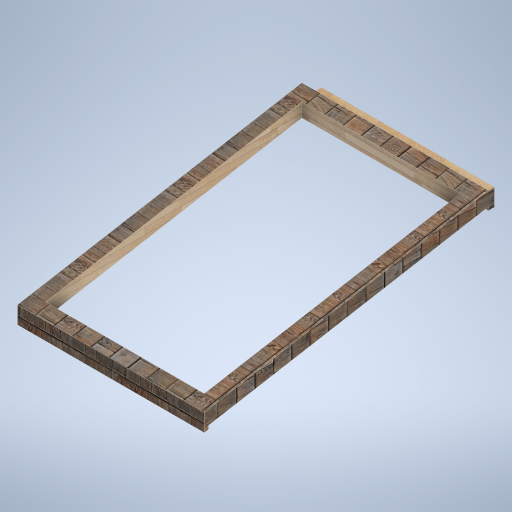
# Autodesk Inventor part: eave_frame_01
Saved by Autodesk Inventor 2024.3 (Build 283343000, 343)
## iProperties
Created: 2024-05-23
Part Number: eave_frame_01
Material: Wood (Maple)
Document SubType Name: Modeling
Designer: Huang
Density: 0.67 g/cm^3
Appearance: Natural Maple - Glossy Dark Tint
Author: Huang
Autodesk Inventor part; units mm, degrees
ref_plane "YZ Plane" through (0, 0, 0) normal (1, 0, 0) x (0, 1, 0)
ref_plane "XZ Plane" through (0, 0, 0) normal (0, 1, 0) x (-1, 0, 0)
sketch "Sketch19" plane through (0, 0, 0) normal (0, 0, 1) x (1, 0, 0)
  line L0 (1200.9555, -1496.1779) -> (1200.9555, 1503.8221)
  line L1 (-4726.1559, 1503.8221) -> (4728.0669, 1503.8221)
  line L2 (4418.0669, -1496.1779) -> (4418.0669, 1503.8221)
  line L3 (1200.9555, 1503.8221) -> (4418.0669, 1503.8221)
  line L4 (1200.9555, 1503.8221) -> (1000.9555, 1503.8221)
  line L5 (1000.9555, 1503.8221) -> (1000.9555, -1496.1779)
  line L6 (2809.5112, 1503.8221) -> (2609.5112, 1503.8221)
  line L7 (2609.5112, 1503.8221) -> (2609.5112, -1496.1779)
  line L8 (2609.5112, -1496.1779) -> (2509.5112, -1496.1779)
  line L9 (2509.5112, -1496.1779) -> (2509.5112, 1503.8221)
  line L10 (1200.9555, -1496.1779) -> (1000.9555, -1496.1779)
  line L11 (1000.9555, 1503.8221) -> (1000.9555, 1353.8221)
  line L12 (1000.9555, 1353.8221) -> (2609.5112, 1353.8221)
  point P0 (0, 0)
  dimension "d29" = 200
  dimension "d30" = 200
  dimension "d31" = 100
  dimension "d32" = 150
  constraints: 26 end point, 6 perpendicular, 5 point on line, 2 coincident, 1 collinear, 1 midpoint
  measures "d29" distance of L3.start L4.end
  measures "d30" distance of L6.start L6.end
  measures "d31" distance of L7.end L8.end
  measures "d32" distance of L4.end L11.end
ref_plane "Work Plane17" through (0, 0, 2500) normal (0, 0, 1) x (1, 0, 0)
sketch "Sketch20" plane through (0, 0, 2500) normal (0, 0, 1) x (1, 0, 0)
  line L0 (-4726.1559, 1503.8221) -> (4728.0669, 1503.8221) projected
  line L1 (1200.9555, -1496.1779) -> (1200.9555, 1503.8221) projected
  line L2 (1000.9555, 1503.8221) -> (1000.9555, -1496.1779) projected
  line L3 (2509.5112, -1496.1779) -> (2509.5112, 1503.8221) projected
  line L4 (2609.5112, 1503.8221) -> (2609.5112, -1496.1779) projected
  line L5 (1000.9555, 1353.8221) -> (2609.5112, 1353.8221) projected
  point P0 (0, 0)
extrude "Extrusion4" add sketch "Sketch19" along normal blind 51 contours L12 L5 L1 L0 | L0 L1 L9 L12 | L9 L1 L7 L12
ref_plane "Work Plane18" through (0, 0, 51) normal (0, 0, 1) x (1, 0, 0)
sketch "Sketch22" plane through (0, 0, 51) normal (0, 0, 1) x (1, 0, 0)
  line L0 (2609.5112, 1503.8221) -> (1000.9555, 1503.8221) projected
  line L1 (1000.9555, 1503.8221) -> (1000.9555, 1353.8221) projected
  line L2 (1000.9555, 1353.8221) -> (2609.5112, 1353.8221) projected
  line L3 (2609.5112, 1353.8221) -> (2609.5112, 1503.8221) projected
  line L4 (1000.9555, 1503.8221) -> (2609.5112, 1503.8221)
  line L5 (2609.5112, 1503.8221) -> (2609.5112, 1353.8221)
  line L6 (2609.5112, 1353.8221) -> (1000.9555, 1353.8221)
  line L7 (1000.9555, 1353.8221) -> (1000.9555, 1503.8221)
  point P0 (0, 0)
  constraints: 8 end point, 2 parallel, 1 horizontal, 1 perpendicular
ref_plane "Work Plane19" through (1000.9555, 1503.8221, 51) normal (-1, 0, 0) x (0, -1, 0)
sketch "Sketch23" plane through (1000.9555, 1503.8221, 51) normal (-1, 0, 0) x (0, -1, 0)
  line L0 (150, 0) -> (0, 0) projected
  line L1 (0, 2449) -> (3000, 2449) projected
  line L2 (0, 0) -> (431.8248, 2449)
  line L3 (0, 0) -> (2486.7798, 0) construction
  line L4 (0, 0) -> (150, 0)
  line L5 (150, 0) -> (0, 0)
  line L6 (150, 0) -> (581.8248, 2449)
  line L7 (150, 0) -> (2636.7798, 0) construction
  line L8 (581.8248, 2449) -> (431.8248, 2449)
  point P0 (1503.8221, -51)
  point P1 (0, 2449)
  dimension "d37" = 80
  dimension "d38" = 80
  constraints: 14 end point, 3 collinear, 2 equal length, 2 horizontal, 2 point on line, 1 coincident
  measures "d37" angle of L3 L2
  measures "d38" angle of L7 L6
sketch "Sketch24" plane through (0, 0, 2500) normal (0, 0, 1) x (1, 0, 0)
  line L0 (1000.9555, 1071.9973) -> (2609.5112, 1071.9973)
  line L1 (1000.9555, 921.9973) -> (2609.5112, 921.9973)
  line L2 (2609.5112, 1071.9973) -> (2609.5112, 921.9973)
  line L3 (1000.9555, 1071.9973) -> (1000.9555, 921.9973)
  point P0 (0, 0)
  constraints: 8 end point, 2 perpendicular
loft "Loft2" add profiles "Sketch24" section 2 edges at (2609.5112, 1428.8221, 51) (1805.2334, 1503.8221, 51) (1000.9555, 1428.8221, 51) (1805.2334, 1353.8221, 51)
sketch "Sketch25" plane through (2609.5112, 1353.8221, 0) normal (1, 0, 0) x (0, 0, -1)
  line L0 (0, 0) -> (0, 150) projected
  line L1 (0, 150) -> (-51, 150) projected
  line L2 (-2500, -281.8248) -> (-51, 150) projected
  line L3 (-2500, -281.8248) -> (-2500, -431.8248) projected
  line L4 (-2500, -431.8248) -> (-51, 0) projected
  line L5 (0, 0) -> (-51, 0) projected
  line L6 (-51, 0) -> (-51, 29.8153)
  line L7 (-51, 0) -> (-21.1847, 0) construction
  line L8 (-51, 29.8153) -> (-2463.779, -395.6227)
  line L9 (-2500, -431.8248) -> (-51, 0) projected
  line L10 (-51, 29.8153) -> (2399, 29.8153) construction
  line L11 (-2463.779, -395.6227) -> (-2463.779, -425.438)
  line L12 (-2463.779, -425.438) -> (-51, 0)
  point P0 (0, -1353.8221)
  point P1 (-2463.779, -425.438)
  point P2 (-51, 0)
  dimension "d43" = 90
  dimension "d44" = 2450
  dimension "d45" = 170
  constraints: 12 end point, 2 coincident, 2 equal length, 2 horizontal, 1 collinear, 1 parallel, 1 point on line, 1 vertical
  measures "d43" angle of L7 L6
  measures "d44" distance of L6.end L8.end
  measures "d45" angle of L8 L10
extrude "Extrusion5" cut sketch "Sketch25" against normal through all contours L4 L11 L8 L6
ref_plane "Work Plane20" through (4728.0669, 1503.8221, 51) normal (0, -1, 0) x (-1, 0, 0)
sketch "Sketch26" plane through (4728.0669, 1503.8221, 51) normal (0, -1, 0) x (-1, 0, 0)
  line L0 (2118.5557, 0) -> (3727.1114, 0) projected
  line L1 (3727.1114, -2449) -> (3727.1114, 0) projected
  line L2 (2118.5557, -2449) -> (2118.5557, 0) projected
  line L3 (3727.1114, -2449) -> (2118.5557, -2449) projected
  line L4 (2118.5557, -2449) -> (2238.5978, -2449)
  line L5 (2238.5978, -2449) -> (2238.5978, -2329)
  line L6 (2238.5978, -2329) -> (2118.5557, -2329)
  line L7 (2118.5557, -2329) -> (2118.5557, -2449)
  line L8 (3727.1114, 0) -> (3607.1114, 0)
  line L9 (3607.1114, 0) -> (3607.1114, -120)
  line L10 (3607.1114, -120) -> (3727.1114, -120)
  line L11 (3727.1114, -120) -> (3727.1114, 0)
  line L12 (3607.1114, -120) -> (2238.5978, -120)
  line L13 (2238.5978, -120) -> (2238.5978, -2329)
  line L14 (2238.5978, -2329) -> (3607.1114, -2329)
  line L15 (3607.1114, -2329) -> (3607.1114, -120)
  point P0 (4728.0669, 51)
  dimension "d49" = 120
  dimension "d50" = 120
  dimension "d51" = 120
  constraints: 24 end point, 6 parallel, 3 horizontal, 3 perpendicular
  measures "d49" distance of L5.end L4.end
  measures "d50" distance of L10.end L9.end
  measures "d51" distance of L9.end L8.end
extrude "Extrusion6" cut sketch "Sketch26" along normal through all contours L15 L14 L13 L12
sketch "Sketch27" plane through (1000.9555, 1503.8221, 0) normal (0, 1, 0) x (1, 0, 0)
  line L0 (1608.5557, 0) -> (0, 0) projected
  line L1 (0, 0) -> (120, 0)
  line L2 (120, 0) -> (120, -51)
  line L3 (0, 0) -> (0, -51) projected
  line L4 (1608.5557, -51) -> (0, -51) projected
  line L5 (0, 0) -> (0, -51)
  line L6 (0, -51) -> (120, -51)
  line L7 (120, -2380) -> (120, -171) projected
  line L8 (0, -2500) -> (0, -51) projected
  point P0 (-1000.9555, 0)
  dimension "d54" = 120
  constraints: 8 end point, 2 perpendicular, 1 point on line
  measures "d54" distance of L0.end L1.end
extrude "Extrusion7" cut sketch "Sketch27" against normal through all
body "Solid2"
